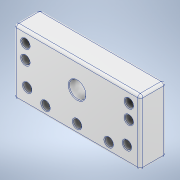
# Autodesk Inventor part: 5213_Bias_TxRx_Relative_Adapter_MPSv2_v1
Saved by Autodesk Inventor 2021 (Build 250183000, 183)
## iProperties
Created: 2020-11-14
Part Number: 5213_Bias_TxRx_Relative_Adapter_MPSv2_v1
Material: Aluminum 6061
Document SubType Name: Modeling
Designer: Admin
Density: 2.7 g/cm^3
Appearance: Aluminum - Flat
Author: Admin
Autodesk Inventor part; units mm, degrees
sketch "Sketch1" plane through (0, 0, 0) normal (0, 0, 1) x (1, 0, 0)
  line L0 (-48.9, 9.525) -> (48.9, 9.525)
  line L1 (48.9, 9.525) -> (48.9, -9.525)
  line L2 (48.9, -9.525) -> (-48.9, -9.525)
  line L3 (-48.9, -9.525) -> (-48.9, 9.525)
  line L4 (-48.9, 9.525) -> (48.9, -9.525) construction
  line L5 (48.9, 9.525) -> (-48.9, -9.525) construction
  line L6 (48.9, 9.525) -> (48.9, 5.525)
  circle A0 centre (-24.45, -2) radius 3.175
  circle A1 centre (0, -2) radius 3.175
  circle A2 centre (24.45, -2) radius 3.175
  line L7 (24.45, -2) -> (39.45, -2) construction
  circle A3 centre (38.5454, 3.1303) radius 3.175
  line L8 (-24.45, -2) -> (-9.45, -2) construction
  circle A4 centre (-38.5454, 3.1303) radius 3.175
  point P0 (0, 0)
  dimension "d0" = 97.8
  dimension "d1" = 19.05
  dimension "d3" = 4
  dimension "d7" = 6.35
  dimension "d8" = 6.35
  dimension "d9" = 6.35
  dimension "d25" = 6.35
  dimension "d28" = 6.35
  constraints: 18 end point, 5 centre point, 3 horizontal, 2 midpoint, 2 parallel, 1 perpendicular, 1 point on line
  measures "d0" distance of L1.end L2.end
  measures "d1" distance of L0.end L1.end
  measures "d3" distance of L0.end L6.end
  measures "d7" diameter of A0
  measures "d8" diameter of A1
  measures "d9" diameter of A2
  measures "d25" diameter of A3
  measures "d28" diameter of A4
ref_plane "Work Plane2" through (0, 0, 0) normal (0, 0, -1) x (-1, 0, 0)
sketch "Sketch2" plane through (0, 0, 0) normal (0, 0, -1) x (-1, 0, 0)
  line L0 (-48.9, 9.525) -> (48.9, 9.525) projected
  line L1 (-48.9, 9.525) -> (48.9, 9.525)
  line L2 (48.9, 9.525) -> (48.9, 30.925)
  line L3 (48.9, 30.925) -> (-48.9, 30.925)
  line L4 (-48.9, 30.925) -> (-48.9, 9.525)
  circle A0 centre (0, -2) radius 2.5 projected
  line L5 (0, -2) -> (0, 9.525)
  line L6 (0, 9.525) -> (0, 20.725)
  circle A1 centre (0, 20.725) radius 6.35
  point P0 (0, 0)
  dimension "d12" = 21.4
  dimension "d13" = 11.2
  dimension "d14" = 12.7
  constraints: 12 end point, 2 parallel, 1 centre point, 1 coincident, 1 horizontal, 1 midpoint, 1 perpendicular, 1 point on line
  measures "d12" distance of L2.end L1.end
  measures "d13" distance of L5.end L6.end
  measures "d14" diameter of A1
extrude "Extrusion2" add sketch "Sketch2" against normal blind 20 contours L4 L3 L2 L0
ref_plane "Work Plane1" through (0, 0, 0) normal (0, 0, -1) x (-1, 0, 0)
sketch "Sketch3" plane through (0, 0, 0) normal (0, 0, -1) x (-1, 0, 0)
  line L0 (-48.9, -9.525) -> (-48.9, 30.925) projected
  line L1 (-48.9, 30.925) -> (48.9, 30.925)
  line L2 (48.9, 30.925) -> (48.9, 40.925)
  line L3 (48.9, 40.925) -> (-48.9, 40.925)
  line L4 (-48.9, 40.925) -> (-48.9, 30.925)
  point P0 (0, 0)
  dimension "d17" = 10
  constraints: 8 end point, 2 parallel, 1 horizontal, 1 perpendicular
  measures "d17" distance of L2.end L1.end
extrude "Extrusion3" add sketch "Sketch3" against normal blind 20
ref_plane "Work Plane3" through (0, 0, 0) normal (0, 0, -1) x (-1, 0, 0)
sketch "Sketch4" plane through (0, 0, 0) normal (0, 0, -1) x (-1, 0, 0)
  circle A0 centre (0, 20.725) radius 6.35 projected
  circle A1 centre (0, 20.725) radius 11.1125
  point P0 (0, 0)
  dimension "d20" = 22.225
  constraints: 1 centre point, 1 coincident
  measures "d20" diameter of A1
extrude "Extrusion4" cut sketch "Sketch4" against normal blind 1.5875
sketch "Sketch5" plane through (0, 0, 0) normal (0, 0, -1) x (-1, 0, 0)
  point P0 (0, 0)
extrude "Extrusion5" add sketch "Sketch1" along normal blind 20
sketch "Sketch6" plane through (0, 0, 0) normal (0, 0, -1) x (-1, 0, 0)
  circle A0 centre (0, 20.725) radius 11.1125 projected
  line L0 (0, 20.725) -> (-40, 20.725)
  circle A1 centre (0, 20.725) radius 6.35 projected
  line L1 (0, 20.725) -> (40, 20.725)
  line L2 (0, 31.8375) -> (-40, 31.8375)
  line L3 (0, 31.8375) -> (40, 31.8375)
  circle A2 centre (-40, 31.8375) radius 3.175
  circle A3 centre (-40, 20.725) radius 3.175
  circle A4 centre (40, 31.8375) radius 3.175
  circle A5 centre (40, 20.725) radius 3.175
  point P0 (0, 0)
  dimension "d31" = 40
  dimension "d32" = 40
  dimension "d33" = 40
  dimension "d34" = 6.35
  dimension "d35" = 6.35
  dimension "d36" = 6.35
  dimension "d37" = 6.35
  constraints: 8 end point, 4 centre point, 4 coincident, 4 horizontal, 1 vertical alignment, 1 other
  measures "d31" distance of L0.start L0.end
  measures "d32" distance of L1.start L1.end
  measures "d33" distance of L2.start L2.end
  measures "d34" diameter of A2
  measures "d35" diameter of A3
  measures "d36" diameter of A4
  measures "d37" diameter of A5
extrude "Extrusion6" cut sketch "Sketch6" against normal blind 20 contours A2 | A3 | A4 | A5
fillet "Fillet1" radius 2 12 edges at (0, 40.925, 0) (48.9, 15.7, 0) (48.9, 15.7, 20) (48.9, 40.925, 10) (-48.9, 40.925, 10) (0, 40.925, 20) (-48.9, 15.7, 20) (-48.9, 15.7, 0) (-48.9, -9.525, 10) (0, -9.525, 20) (0, -9.525, 0) (48.9, -9.525, 10)
fillet "Fillet2" radius 0.5 21 edges at (6.35, 20.725, 20) (-27.625, -2, 20) (-41.7204, 3.1303, 20) (-3.175, -2, 20) (21.275, -2, 20) (35.3704, 3.1303, 20) (43.175, 20.725, 20) (43.175, 31.8375, 20) (-36.825, 20.725, 20) (-36.825, 31.8375, 20) (43.175, 31.8375, 0) (43.175, 20.725, 0) (35.3704, 3.1303, 0) (21.275, -2, 0) (-3.175, -2, 0) (-27.625, -2, 0) (-41.7204, 3.1303, 0) (-36.825, 20.725, 0) (-36.825, 31.8375, 0) (11.1125, 20.725, 0) (6.35, 20.725, 1.5875)
body "Solid1"
